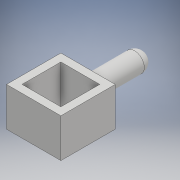
# Autodesk Inventor part: 軸滑塊
Saved by Autodesk Inventor 2017 (Build 210142000, 142)
## iProperties
Part Number: 軸滑塊
Material: 一般
Document SubType Name: Modeling
Designer: Brian
Density: 1 g/cm^3
Appearance: 預設
Author: Brian
Autodesk Inventor part; units mm, degrees
ref_plane "YZ Plane" through (0, 0, 0) normal (1, 0, 0) x (0, 1, 0)
ref_plane "XZ Plane" through (0, 0, 0) normal (0, 1, 0) x (-1, 0, 0)
ref_plane "XY Plane" through (0, 0, 0) normal (0, 0, 1) x (1, 0, 0)
sketch "草圖1" plane through (0, 0, 0) normal (0, 0, 1) x (1, 0, 0)
  line L0 (-5, -5) -> (5, -5)
  line L1 (5, -5) -> (5, 5)
  line L2 (5, 5) -> (-5, 5)
  line L3 (-5, 5) -> (-5, -5)
  line L4 (-5, -5) -> (5, 5) construction
  line L5 (5, -5) -> (-5, 5) construction
  line L6 (-7, 7) -> (7, 7)
  line L7 (7, 7) -> (7, -7)
  line L8 (7, -7) -> (-7, -7)
  line L9 (-7, -7) -> (-7, 7)
  point P0 (0, 0)
  dimension "d0" = 10
  dimension "d1" = 10
  dimension "d2" = 2
  constraints: 20 end point, 4 parallel, 2 midpoint, 2 perpendicular, 1 horizontal, 3 other
  measures "d0" distance of L1.end L2.end
  measures "d1" distance of L0.end L1.end
  measures "d2" distance between parallel lines of L3 L9
extrude "擠出1" add sketch "草圖1" along normal blind 10
sketch "草圖2" plane through (-7, 7, 0) normal (0, 1, 0) x (1, 0, 0)
  line L0 (2, -10) -> (12, -10) projected
  line L1 (12, 0) -> (2, 0) projected
  line L2 (4, -10) -> (9, -10)
  line L3 (9, -10) -> (9, 0)
  line L4 (9, 0) -> (4, 0)
  line L5 (4, 0) -> (4, -10)
  line L6 (14, 0) -> (14, -10) projected
  point P0 (7, 0)
  dimension "d5" = 5
  dimension "d6" = 5
  constraints: 8 end point, 2 parallel, 2 point on line, 1 horizontal, 1 perpendicular
  measures "d5" distance between parallel lines of L5 L3
  measures "d6" distance between parallel lines of L6 L3
extrude "擠出2" add sketch "草圖2" along normal blind 15
sketch "草圖3" plane through (0, 0, 10) normal (0, 0, 1) x (1, 0, 0)
  line L0 (-7, 7) -> (-3, 7) projected
  line L1 (-7, 7) -> (8.7829, 7)
  line L2 (8.7829, 7) -> (8.7829, 28.6907)
  line L3 (8.7829, 28.6907) -> (-7, 28.6907)
  line L4 (-7, 28.6907) -> (-7, 7)
  point P0 (0, 0)
  constraints: 8 end point, 2 parallel, 1 horizontal, 1 perpendicular
extrude "擠出3" cut sketch "草圖3" against normal blind 2.5
sketch "草圖4" plane through (0, 0, 0) normal (0, 0, -1) x (-1, 0, 0)
  line L0 (-2, 7) -> (-7, 7) projected
  line L1 (-3.5131, 7) -> (8.3925, 7)
  line L2 (8.3925, 7) -> (8.3925, 27.422)
  line L3 (8.3925, 27.422) -> (-3.5131, 27.422)
  line L4 (-3.5131, 27.422) -> (-3.5131, 7)
  point P0 (0, 0)
  constraints: 8 end point, 2 parallel, 1 horizontal, 1 perpendicular, 1 point on line
extrude "擠出4" cut sketch "草圖4" against normal blind 2.5
fillet "圓角2" radius 2.5 4 edges at (-3, 14.5, 7.5) (2, 14.5, 7.5) (2, 14.5, 2.5) (-3, 14.5, 2.5)
fillet "圓角3" radius 2.5 3 edges at (-3, 22, 5) (-2.2678, 22, 6.7678) (-0.5, 22, 7.5)
